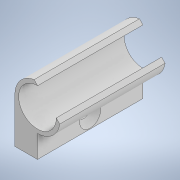
# Autodesk Inventor part: shadeHolderKetchenWindowV2
Saved by Autodesk Inventor 2022 (Build 260153070, 153G)
## iProperties
Created: 2021-02-12
Part Number: shadeHolderKetchenWindowV2
Material: Generic
Document SubType Name: Modeling
Designer: robst
Density: 1 g/cm^3
Appearance: Default
Author: robst
Autodesk Inventor part; units mm, degrees
ref_plane "YZ Plane" through (0, 0, 0) normal (1, 0, 0) x (0, 1, 0)
ref_plane "XZ Plane" through (0, 0, 0) normal (0, 1, 0) x (-1, 0, 0)
ref_plane "XY Plane" through (0, 0, 0) normal (0, 0, 1) x (1, 0, 0)
sketch "Sketch4" plane through (0, 0, 0) normal (0, 0, 1) x (1, 0, 0)
  arc A0 (0.0635, 6.3497) -> (6.3497, 0.0635) centre (0, 0) ccw
  arc A1 (-1.1235, 7.5367) -> (7.5367, -1.1235) centre (0, 0) ccw
  line L0 (0, 0) -> (0, 7.9375) construction
  line L1 (0.0635, 6.3497) -> (6.3497, 0.0635) construction
  line L2 (0.0635, 6.3497) -> (-1.1235, 7.5367)
  line L3 (6.3497, 0.0635) -> (7.5367, -1.1235)
  circle A2 centre (0, 0) radius 6.35
  dimension "d10" = 12.7
  dimension "d11" = 1.27
  dimension "d12" = 45
  dimension "d13" = 8.89
  constraints: 8 end point, 4 point on circle, 3 centre point, 3 coincident, 1 collinear, 1 concentric, 1 point on line, 1 vertical
  measures "d10" diameter of A0
  measures "d11" radial gap between concentric circles of A1 A0
  measures "d12" angle of L1 L0
  measures "d13" distance of L1.start L1.end
extrude "Extrusion3" add sketch "Sketch4" along normal mid plane 35.56 contours A0 L3 A1 L2
sketch "Sketch5" plane through (0, 0, 0) normal (0, 0, 1) x (1, 0, 0)
  arc A0 (-1.1235, 7.5367) -> (7.5367, -1.1235) centre (0, 0) ccw projected
  line L0 (-7.62, 0) -> (-7.62, -15.24)
  line L1 (-7.62, -15.24) -> (0, -15.24)
  line L2 (0, -15.24) -> (0, -7.62)
  circle A1 centre (0, 0) radius 7.9375
  dimension "d16" = 7.62
  constraints: 6 end point, 2 perpendicular, 2 point on circle, 1 centre point, 1 coincident, 1 tangent, 1 vertical
  measures "d16" distance from line of L2.end L1
extrude "Extrusion4" add sketch "Sketch5" along normal mid plane 35.56 contours A0 L2 A1 L0 | A1 L2 L1 L0 picked at (-7.3048, -2.4081)
sketch "Sketch6" plane through (0, -15.24, 17.78) normal (1, 0, 0) x (0, 0, -1)
  line L0 (0, 7.62) -> (35.56, 7.62) projected
  line L1 (35.56, 7.62) -> (35.56, 0) projected
  line L2 (0, 0) -> (35.56, 0) projected
  line L3 (0, 0) -> (0, 7.62) projected
  line L4 (17.78, 0) -> (17.78, 7.62) construction
  point P0 (17.78, 15.24)
  point P1 (17.78, 3.81)
  dimension "d30" = 3.81
  dimension "d31" = 0
  constraints: 2 end point, 2 midpoint
  measures "d30" distance from line of point (17.78, 3.81) L2
  measures "d31" distance from line of point (17.78, 3.81) L4
hole "Hole1" at (0, -11.43, 0) direction (-1, 0, 0) diameter 3.5052 end through all countersink diameter 7.112 countersink angle 82
sketch "Sketch10" plane through (-7.62, -15.24, 17.78) normal (0, -1, 0) x (1, 0, 0)
  line L0 (0, -35.56) -> (0, 0) projected
  line L1 (7.62, -35.56) -> (0, -35.56) projected
  line L2 (7.62, 0) -> (7.62, -35.56) projected
  line L3 (0, 0) -> (7.62, 0) projected
  line L4 (3.81, -35.56) -> (3.81, 0) construction
  line L5 (6.096, -30.4401) -> (6.096, -31.2292)
  line L6 (6.096, -31.2292) -> (3.9693, -32.9002)
  line L7 (3.9693, -32.9002) -> (4.2694, -33.167)
  line L8 (4.2694, -33.167) -> (6.096, -33.167)
  line L9 (6.096, -33.167) -> (6.096, -33.7746)
  line L10 (6.096, -33.7746) -> (1.524, -33.7746)
  line L11 (1.524, -33.7746) -> (1.524, -33.167)
  line L12 (1.524, -33.167) -> (3.6247, -33.167)
  line L13 (3.6247, -33.167) -> (1.524, -31.2922)
  line L14 (1.524, -31.2922) -> (1.524, -30.5512)
  line L15 (1.524, -30.5512) -> (3.5655, -32.4445)
  line L16 (3.5655, -32.4445) -> (6.096, -30.4401)
  line L17 (1.524, -24.9529) -> (6.096, -26.1015)
  line L18 (6.096, -26.1015) -> (6.096, -26.7832)
  line L19 (6.096, -26.7832) -> (2.3021, -27.7132)
  line L20 (2.3021, -27.7132) -> (6.096, -28.6172)
  line L21 (6.096, -28.6172) -> (6.096, -29.2915)
  line L22 (6.096, -29.2915) -> (1.524, -30.4586)
  line L23 (1.524, -30.4586) -> (1.524, -29.8324)
  line L24 (1.524, -29.8324) -> (5.3142, -28.9136)
  line L25 (5.3142, -28.9136) -> (1.524, -28.0022)
  line L26 (1.524, -28.0022) -> (1.524, -27.3834)
  line L27 (1.524, -27.3834) -> (5.3587, -26.4646)
  line L28 (5.3587, -26.4646) -> (1.524, -25.5494)
  line L29 (1.524, -25.5494) -> (1.524, -24.9529)
  line L30 (1.524, -21.0923) -> (6.096, -22.6669)
  line L31 (6.096, -22.6669) -> (6.096, -23.3227)
  line L32 (6.096, -23.3227) -> (1.524, -24.8974)
  line L33 (1.524, -24.8974) -> (1.524, -24.2453)
  line L34 (1.524, -24.2453) -> (5.3216, -22.9781)
  line L35 (5.3216, -22.9781) -> (1.524, -21.711)
  line L36 (1.524, -21.711) -> (1.524, -21.0923)
  spline S0 degree 2 poles (3.81, -17.8874) (5.0401, -17.8874) (6.1923, -18.6025) (6.1923, -19.3472) knots 0 0 0 1 2 2 2
  spline S1 degree 2 poles (6.1923, -19.3472) (6.1923, -20.1031) (5.0178, -20.8107) (3.8137, -20.8107) knots 0 0 0 1 2 2 2
  spline S2 degree 2 poles (3.8137, -20.8107) (2.5762, -20.8107) (1.4314, -20.0956) (1.4314, -19.3472) knots 0 0 0 1 2 2 2
  spline S3 degree 2 poles (1.4314, -19.3472) (1.4314, -18.5951) (2.617, -17.8874) (3.81, -17.8874) knots 0 0 0 1 2 2 2
  spline S4 degree 2 poles (5.2031, -18.6729) (4.9771, -18.584) (4.2805, -18.5099) (3.81, -18.5099) knots 0 0 0 1 2 2 2
  spline S5 degree 2 poles (3.81, -18.5099) (3.3395, -18.5099) (2.6466, -18.584) (2.4132, -18.6766) knots 0 0 0 1 2 2 2
  spline S6 degree 2 poles (2.4132, -18.6766) (2.1798, -18.7692) (1.939, -19.0916) (1.939, -19.3472) knots 0 0 0 1 2 2 2
  spline S7 degree 2 poles (1.939, -19.3472) (1.939, -19.6029) (2.1798, -19.9326) (2.4206, -20.0289) knots 0 0 0 1 2 2 2
  spline S8 degree 2 poles (2.4206, -20.0289) (2.654, -20.1216) (3.3654, -20.1883) (3.8137, -20.1883) knots 0 0 0 1 2 2 2
  spline S9 degree 2 poles (3.8137, -20.1883) (4.2954, -20.1883) (4.94, -20.129) (5.192, -20.0327) knots 0 0 0 1 2 2 2
  spline S10 degree 2 poles (5.192, -20.0327) (5.4291, -19.9437) (5.6847, -19.614) (5.6847, -19.3472) knots 0 0 0 1 2 2 2
  spline S11 degree 2 poles (5.6847, -19.3472) (5.6847, -19.0953) (5.4439, -18.7655) (5.2031, -18.6729) knots 0 0 0 1 2 2 2
  line L37 (6.096, -14.4825) -> (6.096, -17.3021)
  line L38 (6.096, -17.3021) -> (5.4476, -17.3021)
  spline S12 degree 2 poles (5.4476, -17.3021) (5.1623, -16.9982) (4.6325, -16.4573) (4.3472, -16.198) knots 0 0 0 1 2 2 2
  spline S13 degree 2 poles (4.3472, -16.198) (3.7729, -15.6755) (3.0838, -15.2939) (2.717, -15.2939) knots 0 0 0 1 2 2 2
  spline S14 degree 2 poles (2.717, -15.2939) (2.5244, -15.2939) (2.2354, -15.4125) (2.1427, -15.5199) knots 0 0 0 1 2 2 2
  spline S15 degree 2 poles (2.1427, -15.5199) (2.0501, -15.6274) (1.9575, -15.909) (1.9575, -16.0794) knots 0 0 0 1 2 2 2
  spline S16 degree 2 poles (1.9575, -16.0794) (1.9575, -16.2424) (2.039, -16.5759) (2.102, -16.7278) knots 0 0 0 1 2 2 2
  spline S17 degree 2 poles (2.102, -16.7278) (2.1539, -16.8574) (2.3021, -17.0983) (2.3539, -17.1724) knots 0 0 0 1 2 2 2
  line L39 (2.3539, -17.1724) -> (2.3539, -17.2057)
  line L40 (2.3539, -17.2057) -> (1.7018, -17.2057)
  spline S18 degree 2 poles (1.7018, -17.2057) (1.6092, -17.0168) (1.4277, -16.3387) (1.4277, -16.0349) knots 0 0 0 1 2 2 2
  spline S19 degree 2 poles (1.4277, -16.0349) (1.4277, -15.394) (2.1057, -14.6715) (2.6837, -14.6715) knots 0 0 0 1 2 2 2
  spline S20 degree 2 poles (2.6837, -14.6715) (2.9541, -14.6715) (3.4062, -14.7975) (3.5988, -14.9086) knots 0 0 0 1 2 2 2
  spline S21 degree 2 poles (3.5988, -14.9086) (3.7989, -15.0198) (4.1916, -15.3421) (4.3806, -15.5199) knots 0 0 0 1 2 2 2
  spline S22 degree 2 poles (4.3806, -15.5199) (4.6955, -15.8089) (5.3698, -16.5166) (5.5662, -16.7278) knots 0 0 0 1 2 2 2
  line L41 (5.5662, -16.7278) -> (5.5662, -14.4825)
  line L42 (5.5662, -14.4825) -> (6.096, -14.4825)
  line L43 (4.3732, -12.1965) -> (4.3732, -13.9268)
  line L44 (4.3732, -13.9268) -> (3.8174, -13.9268)
  line L45 (3.8174, -13.9268) -> (3.8174, -12.1965)
  line L46 (3.8174, -12.1965) -> (4.3732, -12.1965)
  spline S23 degree 2 poles (2.9023, -8.5693) (3.1987, -8.5693) (3.7322, -8.7805) (3.9174, -8.9695) knots 0 0 0 1 2 2 2
  spline S24 degree 2 poles (3.9174, -8.9695) (4.1509, -9.2066) (4.3917, -9.8475) (4.3917, -10.3366) knots 0 0 0 1 2 2 2
  line L47 (4.3917, -10.3366) -> (4.3917, -10.8516)
  line L48 (4.3917, -10.8516) -> (6.096, -10.8516)
  line L49 (6.096, -10.8516) -> (6.096, -11.4592)
  line L50 (6.096, -11.4592) -> (1.524, -11.4592)
  line L51 (1.524, -11.4592) -> (1.524, -10.3107)
  spline S25 degree 2 poles (1.524, -10.3107) (1.524, -9.9031) (1.6574, -9.3325) (1.8093, -9.1139) knots 0 0 0 1 2 2 2
  spline S26 degree 2 poles (1.8093, -9.1139) (1.9834, -8.8583) (2.5207, -8.5693) (2.9023, -8.5693) knots 0 0 0 1 2 2 2
  spline S27 degree 2 poles (2.9208, -9.2029) (2.6837, -9.2029) (2.3354, -9.3659) (2.2242, -9.5326) knots 0 0 0 1 2 2 2
  spline S28 degree 2 poles (2.2242, -9.5326) (2.1279, -9.6771) (2.0501, -10.0624) (2.0501, -10.3477) knots 0 0 0 1 2 2 2
  line L52 (2.0501, -10.3477) -> (2.0501, -10.8516)
  line L53 (2.0501, -10.8516) -> (3.873, -10.8516)
  line L54 (3.873, -10.8516) -> (3.873, -10.4366)
  spline S29 degree 2 poles (3.873, -10.4366) (3.873, -10.0661) (3.7544, -9.6104) (3.5988, -9.4622) knots 0 0 0 1 2 2 2
  spline S30 degree 2 poles (3.5988, -9.4622) (3.4617, -9.3251) (3.1394, -9.2029) (2.9208, -9.2029) knots 0 0 0 1 2 2 2
  line L55 (1.524, -4.6753) -> (6.096, -6.25)
  line L56 (6.096, -6.25) -> (6.096, -6.9058)
  line L57 (6.096, -6.9058) -> (1.524, -8.4804)
  line L58 (1.524, -8.4804) -> (1.524, -7.8283)
  line L59 (1.524, -7.8283) -> (5.3216, -6.5612)
  line L60 (5.3216, -6.5612) -> (1.524, -5.2941)
  line L61 (1.524, -5.2941) -> (1.524, -4.6753)
  line L62 (6.096, -1.7261) -> (6.096, -3.9566)
  line L63 (6.096, -3.9566) -> (5.6292, -3.9566)
  line L64 (5.6292, -3.9566) -> (5.6292, -3.1266)
  line L65 (5.6292, -3.1266) -> (2.5651, -3.1266)
  line L66 (2.5651, -3.1266) -> (2.5651, -3.9566)
  line L67 (2.5651, -3.9566) -> (2.1464, -3.9566)
  spline S31 degree 2 poles (2.1464, -3.9566) (2.1464, -3.486) (1.8797, -3.0414) (1.5092, -3.0118) knots 0 0 0 1 2 2 2
  line L68 (1.5092, -3.0118) -> (1.5092, -2.5375)
  line L69 (1.5092, -2.5375) -> (5.6292, -2.5375)
  line L70 (5.6292, -2.5375) -> (5.6292, -1.7261)
  line L71 (5.6292, -1.7261) -> (6.096, -1.7261)
  point P0 (7.62, -17.78)
  constraints: 2 end point, 2 midpoint, 1 vertical
extrude "Text" cut sketch "Sketch10" against normal blind 1.143 contours L5 L6 L7 L8 L9 L10 L11 L12 L13 L14 L15 L16 | L17 L18 L19 L20 L21 L22 L23 L24 L25 L26 L27 L28 L29 | L30 L31 L32 L33 L34 L35 L36 | S0 S1 S2 S3 | L37 L38 S12 S13 S14 S15 S16 S17 L39 L40 S18 S19 S20 S21 S22 L41 L42 | L43 L44 L45 L46 | S23 S24 L47 L48 L49 L50 L51 S25 S26 | L55 L56 L57 L58 L59 L60 L61 | L62 L63 L64 L65 L66 L67 S31 L68 L69 L70 L71
equation "\"d10\" = shadeDiameter"
equation "\"d11\" = shadeHolderWallThickness"
equation "\"d13\" = openingForShade"
equation "\"d14\" = partWidth"
equation "\"d16\" = flatBelowShade"
equation "\"d17\" = partWidth"
equation "\"d30\" = holeHeightAboveBottom"
equation "\"d28\" = textDepth"
equation "\"shadeDiameter\" = 12.7"
equation "\"partWidth\" = 35.56"
equation "\"backThickness\" = 1.905"
equation "\"backHeight\" = 25.4"
equation "\"cutTiltAngle\" = 45deg"
equation "\"flatBelowShade\" = 7.62"
equation "\"shadeHolderWallThickness\" = 1.27"
equation "\"openingForShade\" = 8.89"
equation "\"textDepth\" = 1.143"
equation "\"holeHeightAboveBottom\" = 3.81"
body "Solid2"
